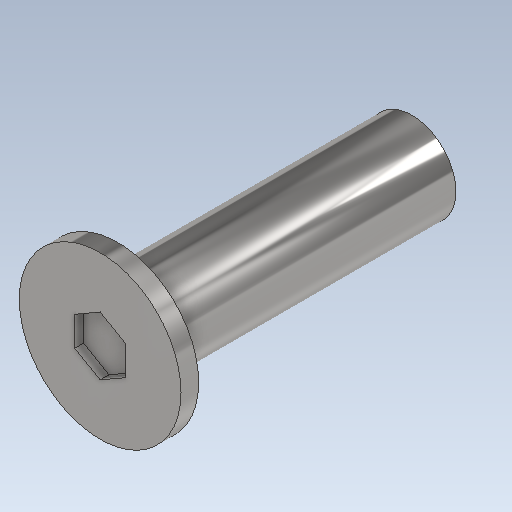
# Autodesk Inventor part: M3極低頭ネジ　10
Saved by Autodesk Inventor 2020 (Build 240168000, 168)
## iProperties
Created: 2020-03-24
Part Number: M3極低頭ネジ　10
Material: 鋼、高強度、低合金
Document SubType Name: Modeling
Designer: happy
Density: 7.85 g/cm^3
Appearance: 鋼 - つや出し
Mass: 0.660667 g
Surface Area: 1.53932 cm^2
Volume: 0.0841614 cm^3
Author: happy
Autodesk Inventor part; units mm, degrees
ref_plane "YZ Plane" through (0, 0, 0) normal (1, 0, 0) x (0, 1, 0)
ref_plane "XZ Plane" through (0, 0, 0) normal (0, 1, 0) x (-1, 0, 0)
ref_plane "XY Plane" through (0, 0, 0) normal (0, 0, 1) x (1, 0, 0)
sketch "スケッチ1" plane through (0, 0, 0) normal (0, 0, 1) x (1, 0, 0)
  circle A0 centre (0, 0) radius 1.5
  dimension "d0" = 3
  constraints: 1 centre point, 1 coincident
  measures "d0" diameter of A0
extrude "押し出し1" add sketch "スケッチ1" along normal blind 10
sketch "スケッチ2" plane through (0, 0, 10) normal (0, 0, 1) x (1, 0, 0)
  circle A0 centre (0, 0) radius 2.75
  dimension "d3" = 5.5
  constraints: 1 centre point, 1 coincident
  measures "d3" diameter of A0
extrude "押し出し2" add sketch "スケッチ2" along normal blind 0.6
sketch "スケッチ3" plane through (0, 0, 10.6) normal (0, 0, 1) x (1, 0, 0)
  line L0 (0, -1) -> (-0.866, -0.5)
  line L1 (-0.866, -0.5) -> (-0.866, 0.5)
  line L2 (-0.866, 0.5) -> (0, 1)
  line L3 (0, 1) -> (0.866, 0.5)
  line L4 (0.866, 0.5) -> (0.866, -0.5)
  line L5 (0.866, -0.5) -> (0, -1)
  circle A0 centre (0, 0) radius 2.75 projected
  dimension "d13" = 1
  constraints: 12 end point, 1 coincident, 1 vertical, 13 other
  measures "d13" distance of point (0, 0) L2.end
extrude "押し出し3" cut sketch "スケッチ3" against normal blind 0.3 contours L0 L1 L2 L3 L4 L5
